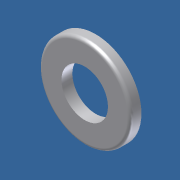
# Autodesk Inventor part: HW-00039
Saved by Autodesk Inventor 2012 (Build 160160000, 160)
## iProperties
Created: 2008-05-01
Part Number: HW-00039
Document SubType Name: Modeling
Designer: dfoster
Density: 1 g/cm^3
Description: Washer, Flat 5/16"
Mass: 0.435823 g
Surface Area: 6.1717 cm^2
Volume: 0.435823 cm^3
Material: Default
Title: Washer, Flat 1/4"
Author: dfoster
Autodesk Inventor part; units mm, degrees
ref_plane "YZ Plane" through (0, 0, 0) normal (1, 0, 0) x (0, 1, 0)
ref_plane "XZ Plane" through (0, 0, 0) normal (0, 1, 0) x (-1, 0, 0)
ref_plane "XY Plane" through (0, 0, 0) normal (0, 0, 1) x (1, 0, 0)
sketch "Sketch1" plane through (0, 0, 0) normal (0, 0, 1) x (1, 0, 0)
  circle A0 centre (0, 0) radius 8.763
  circle A1 centre (0, 0) radius 4.445
  dimension "d0" = 17.526
  dimension "d1" = 8.89
  constraints: 2 centre point, 1 coincident
  measures "d0" diameter of A0
  measures "d1" diameter of A1
extrude "Extrusion1" add sketch "Sketch1" along normal blind 2.0828
fillet "Fillet1" radius 0.635 1 edges at (-8.763, 0, 2.0828)
body "Solid1"
